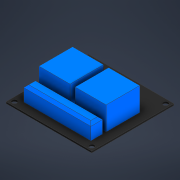
# Autodesk Inventor part: Relais
Saved by Autodesk Inventor 2021 (Build 250183000, 183)
## iProperties
Created: 2020-12-16
Part Number: Relais
Material: Generisch
Document SubType Name: Modeling
Designer: laure
Density: 1 g/cm^3
Appearance: Vorgabe
Author: laure
Autodesk Inventor part; units mm, degrees
ref_plane "YZ Plane" through (0, 0, 0) normal (1, 0, 0) x (0, 1, 0)
ref_plane "XZ Plane" through (0, 0, 0) normal (0, 1, 0) x (-1, 0, 0)
ref_plane "XY Plane" through (0, 0, 0) normal (0, 0, 1) x (1, 0, 0)
sketch "Skizze1" plane through (0, 0, 0) normal (0, 1, 0) x (-1, 0, 0)
  line L0 (25.5, -24.5) -> (-25.5, -24.5)
  line L1 (-25.5, -24.5) -> (-25.5, 24.5)
  line L2 (-25.5, 24.5) -> (25.5, 24.5)
  line L3 (25.5, 24.5) -> (25.5, -24.5)
  line L4 (0, -34.3) -> (0, 34.3) projected
  line L5 (35.7, 0) -> (-35.7, 0) projected
  circle A0 centre (23, -22) radius 1.5
  circle A1 centre (-23, -22) radius 1.5
  circle A2 centre (23, 22) radius 1.5
  circle A3 centre (-23, 22) radius 1.5
  line L6 (20, 12.5) -> (-20, 12.5)
  line L7 (-20, 12.5) -> (-20, 19.5)
  line L8 (-20, 19.5) -> (20, 19.5)
  line L9 (20, 19.5) -> (20, 12.5)
  line L10 (20, 10.3942) -> (1.5, 10.3942)
  line L11 (1.5, 10.3942) -> (1.5, -9.6058)
  line L12 (1.5, -9.6058) -> (20, -9.6058)
  line L13 (20, -9.6058) -> (20, 10.3942)
  line L14 (-20, 10.3942) -> (-1.5, 10.3942)
  line L15 (-1.5, 10.3942) -> (-1.5, -9.6058)
  line L16 (-1.5, -9.6058) -> (-20, -9.6058)
  line L17 (-20, -9.6058) -> (-20, 10.3942)
  point P0 (0, 0)
  dimension "d0" = 51
  dimension "d1" = 49
  dimension "d2" = 3
  dimension "d3" = 2.5
  dimension "d4" = 2.5
  dimension "d5" = 7
  dimension "d6" = 5
  dimension "d7" = 40
  dimension "d8" = 18.5
  dimension "d9" = 20
  constraints: 32 end point, 7 symmetric about line, 6 parallel, 4 centre point, 3 horizontal, 3 perpendicular, 6 other
  measures "d0" distance of L1.end L2.end
  measures "d1" distance of L0.end L1.end
  measures "d2" diameter of A0
  measures "d3" distance from line of L0 A0.centre
  measures "d4" distance from line of L3 A0.centre
  measures "d5" distance between parallel lines of L6 L8
  measures "d6" distance between parallel lines of L8 L2
  measures "d7" distance between parallel lines of L7 L9
  measures "d8" distance of L12.end L11.end
  measures "d9" distance of L11.end L10.end
extrude "Extrusion1" add sketch "Skizze1" along normal blind 1
extrude "Extrusion2" add sketch "Skizze1" along normal blind 10 contours L6 L7 L8 L4 | L4 L8 L9 L6
extrude "Extrusion3" add sketch "Skizze1" along normal blind 15 contours L13 L12 L11 L5 | L5 L11 L10 L13 | L15 L16 L17 L5 | L5 L17 L14 L15
chamfer "Fase1" distance 1.5 angle 45 4 edges at (0, 10, 19.5) (20, 10, 16) (0, 10, 12.5) (-20, 10, 16)
